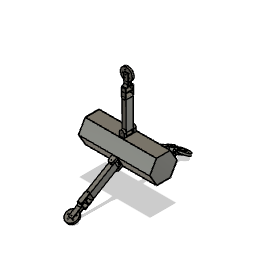
fp1 v5 (Autodesk Fusion 360 design; units mm, degrees)
Autodesk Fusion 360 part; units mm, degrees
sketch "Sketch1" plane through (0, 0, 0) normal (1, 0, 0) x (0, 0, -1)
  line L0 (577.3417, 3.1408) -> (285.9508, 501.563)
  line L1 (285.9508, 501.563) -> (-291.3909, 498.4222)
  line L2 (-291.3909, 498.4222) -> (-577.3417, -3.1408)
  line L3 (-577.3417, -3.1408) -> (-285.9508, -501.563)
  line L4 (-285.9508, -501.563) -> (291.3909, -498.4222)
  line L5 (291.3909, -498.4222) -> (577.3417, 3.1408)
  dimension "d1" = 500
  measures "d1" distance of origin L1
extrude "Extrude1" add sketch "Sketch1" along normal mid plane 3000 makes body 1
copy_body "Body->Comp1" bodies 1 removing the originals makes body 2 in component "old_component"
sketch "Sketch2" plane through (0, 499.9926, 2.72) normal (0, 0.999985, 0.00544) x (1, 0, 0)
  line L0 (-1500, -288.6751) -> (1500, -288.6751)
  line L1 (1500, -288.6751) -> (1500, 288.6751)
  line L2 (1500, 288.6751) -> (-1500, 288.6751)
  line L3 (-1500, 288.6751) -> (-1500, -288.6751)
  line L4 (100, 250) -> (-100, 250)
  line L5 (-100, 250) -> (-100, -250)
  line L6 (-100, -250) -> (100, -250)
  line L7 (100, -250) -> (100, 250)
  line L8 (100, 250) -> (-100, -250) construction
  line L9 (-100, 250) -> (100, -250) construction
  dimension "d4" = 200
  dimension "d5" = 500
  constraint horizontal L4
  constraint perpendicular L4 L5
  constraint parallel L4 L6
  constraint parallel L5 L7
  constraint coincident L8 origin
  constraint coincident L9 origin
  measures "d4" distance of L5.end L6.end
  measures "d5" distance of L4.end L5.end
extrude "Extrude2" add sketch "Sketch2" along normal blind 40 separate body contours L4 L5 L6 L7 makes body 3
sketch "Sketch3" plane through (0, -1.36, 249.9963) normal (0, -0.00544, 0.999985) x (1, 0, 0)
  line L0 (-100, 500) -> (100, 500)
  line L1 (100, 500) -> (100, 540)
  line L2 (100, 540) -> (-100, 540)
  line L3 (-100, 540) -> (-100, 500)
  line L4 (-100, 540) -> (-100, 550)
  line L5 (-100, 550) -> (-100, 650)
  line L6 (100, 540) -> (100, 650)
  circle A0 centre (0, 650) radius 100
  dimension "d8" = 100
  constraint coincident L2.end L3.start
  constraint perpendicular L2 L4
  constraint perpendicular L2 L5
  constraint coincident L1.end L2.start
  constraint perpendicular L2 L6
  constraint coincident L6.end A0
  constraint tangent L6 A0
  measures "d8" distance of L4.end L5.end
extrude "Extrude3" add sketch "Sketch3" against normal blind 500 contours L2 L4 L5 L6 A0 | A0 bodies 3
ref_plane "WorkPlane1" through (0, 624.9908, 3.4) normal (0, 0.00544, -0.999985) x (-1, 0, 0)
sketch "Sketch4" plane through (0, 624.9908, 3.4) normal (0, 0.00544, -0.999985) x (-1, 0, 0)
  arc A0 (100, 25) -> (-100, 25) centre (0, 25) ccw
  line L0 (100, -125) -> (100, 25)
  line L1 (-100, -125) -> (-100, 25)
  line L2 (1500, -125) -> (-1500, -125)
  line L3 (100, -92.0864) -> (-100, -92.0864)
  constraint coincident L0 L3.start
  constraint perpendicular L0 L3
extrude "Extrude4" cut sketch "Sketch4" along normal mid plane 300 contours A0 L0 L1 L3 bodies 3
move_body "Move1" bodies 3 to x (1, 0, 0) y (0, 1, 0) z (0, 0, 1) at (0, 303.2924, 52.7154)
copy_body "Body->Comp2" bodies 3 removing the originals makes body 4 in component "old_component (1)"
sketch "Sketch5" plane through (0, -0.816, 149.9978) normal (0, 0.00544, -0.999985) x (-1, 0, 0)
  arc A0 (100, 650) -> (-100, 650) centre (0, 650) ccw
  line L0 (-100, 650) -> (-100, 532.9136)
  line L1 (-100, 532.9136) -> (100, 532.9136)
  line L2 (100, 532.9136) -> (100, 650)
  line L3 (85, 650) -> (85, 1850)
  arc A1 (85, 1850) -> (-85, 1850) centre (0, 1850) ccw
  line L4 (-85, 1850) -> (-85, 650)
  arc A2 (-85, 650) -> (85, 650) centre (0, 650) ccw
  line L5 (0, 650) -> (0, 1850) construction
  circle A3 centre (0, 650) radius 10
  circle A4 centre (0, 1850) radius 10
  dimension "d18" = 170
  dimension "d19" = 20
  dimension "d20" = 20
  constraint tangent L3 A1
  constraint tangent A1 L4
  constraint parallel L3 L4
  constraint tangent L4 A2
  constraint tangent L3 A2
  constraint vertical L5
  constraint coincident A0.centre A2.centre
  constraint concentric A0 A3
  constraint concentric A1 A4
  measures "d18" diameter of A1
  measures "d19" diameter of A3
  measures "d20" diameter of A4
extrude "Extrude1'" add sketch "Sketch5" along normal blind 300 separate body contours A0 L3 L4 A2 | A0 L3 A1 L4 makes body 5 in component "old_component (2)"
extrude "Extrude1''" cut sketch "Sketch5" along normal blind -120 and the other way blind -550 contours A3 sketch seen with x (1, 0, 0) y (0, 1, 0) z (0, 0, 1) at (0, 303.2924, 52.7154) bodies 4 in component "old_component (1)"
move_body "Move1'" bodies 5 to x (1, 0, 0) y (0, 1, 0) z (0, 0, 1) at (0, 399.9941, 2.176) in component "old_component (2)"
sketch "Sketch6" plane through (-85, 0, 0) normal (-1, 0, 0) x (0, 0, 1)
  line L0 (153.5338, 649.1744) -> (160.0618, 1849.1566)
  line L1 (160.0618, 1849.1566) -> (-139.9337, 1850.7886)
  line L2 (-139.9337, 1850.7886) -> (-146.4618, 650.8064)
  line L3 (-146.4618, 650.8064) -> (153.5338, 649.1744)
  line L4 (-140.075, 1824.8159) -> (-160.0747, 1824.9247)
  line L5 (-160.0747, 1824.9247) -> (-157.7355, 2254.9184)
  line L6 (-137.627, 2274.8093) -> (-127.6271, 2274.7549)
  line L7 (-57.2474, 2344.373) -> (-54.9082, 2774.3667)
  line L8 (-137.7358, 2254.8096) -> (-37.7373, 2254.2655)
  line L9 (-37.7373, 2254.2655) -> (-34.9085, 2774.2579)
  line L10 (-34.9085, 2774.2579) -> (-54.9082, 2774.3667)
  line L11 (159.9206, 1823.1839) -> (179.9203, 1823.0751)
  line L12 (179.9203, 1823.0751) -> (182.2595, 2253.0687)
  line L13 (162.3686, 2273.1772) -> (152.3687, 2273.2316)
  line L14 (82.7506, 2343.6114) -> (85.0898, 2773.6051)
  line L15 (162.2598, 2253.1775) -> (62.2612, 2253.7215)
  line L16 (62.2612, 2253.7215) -> (65.0901, 2773.7139)
  line L17 (65.0901, 2773.7139) -> (85.0898, 2773.6051)
  line L18 (161.4189, 2098.6138) -> (-138.5766, 2100.2458)
  line L19 (-138.6957, 2078.3625) -> (161.2999, 2076.7305)
  line L20 (159.9206, 1823.1839) -> (161.2999, 2076.7305)
  line L21 (161.4189, 2098.6138) -> (162.2598, 2253.1775)
  line L22 (-140.075, 1824.8159) -> (-138.6957, 2078.3625)
  line L23 (-138.5766, 2100.2458) -> (-137.7358, 2254.8096)
  arc A0 (82.7506, 2343.6114) -> (152.3687, 2273.2316) centre (152.7495, 2343.2306) ccw
  arc A1 (-127.6271, 2274.7549) -> (-57.2474, 2344.373) centre (-127.2463, 2344.7538) ccw
  line L24 (182.2595, 2253.0687) -> (162.3686, 2273.1772)
  line L25 (-157.7355, 2254.9184) -> (-137.627, 2274.8093)
  point P0 (-157.6267, 2274.9181)
  point P1 (-57.6282, 2274.3741)
  point P2 (182.3683, 2273.0684)
  point P3 (82.3698, 2273.6124)
  dimension "d47" = 20
  dimension "d48" = 450
  dimension "d49" = 100
  dimension "d50" = 500
  dimension "d52" = 20
  dimension "d53" = 450
  dimension "d54" = 100
  dimension "d55" = 500
  dimension "d57" = 70
  dimension "d58" = 20
  dimension "d59" = 20
  dimension "d60" = 20
  dimension "d61" = 20
  constraint coincident L2 L4.start
  constraint perpendicular L2 L4
  constraint perpendicular L4 L5
  constraint perpendicular L2 L6
  constraint perpendicular L6 L7
  constraint perpendicular L7 L10
  constraint coincident L0 L11.start
  constraint perpendicular L0 L11
  constraint perpendicular L8 L12
  constraint perpendicular L12 L13
  constraint perpendicular L10 L14
  constraint perpendicular L14 L17
  constraint coincident L18.start L20
  constraint coincident L18.end L22
  constraint perpendicular L18 L22
  constraint perpendicular L19 L20
  constraint collinear L20 L21
  constraint collinear L22 L23
  constraint coincident P3 L13
  constraint coincident P3 L14
  constraint tangent L13 A0
  constraint tangent L14 A0
  constraint coincident P1 L6
  constraint coincident P1 L7
  constraint tangent L6 A1
  constraint tangent L7 A1
  constraint equal A0 A1
  constraint coincident P2 L12
  constraint coincident P2 L13
  constraint coincident P0 L5
  constraint coincident P0 L6
  measures "d47" distance of L4.start L4.end
  measures "d48" distance of L4.end P0
  measures "d49" distance of P0 P1
  measures "d50" distance of P1 L7.end
  measures "d52" distance of L11.start L11.end
  measures "d53" distance of L11.end P2
  measures "d54" distance of P2 P3
  measures "d55" distance of P3 L14.end
  measures "d57" radius of A0
  measures "d58" distance of P2 L12.end
  measures "d59" distance of P2 L13.start
  measures "d60" distance of P0 L5.end
  measures "d61" distance of P0 L6.start
ref_plane "WorkPlane2" through (0, 1249.9815, 6.8) normal (0, -0.00544, 0.999985) x (1, 0, 0)
extrude "Extrude1'''" add sketch "Sketch6" against normal blind 170 separate body contours L0 L2 L4 L5 L6 L7 L8 L9 L10 L11 L12 L13 L14 L15 L16 L17 L18 L19 L20 L21 L22 L23 A0 A1 L24 L25 makes body 6 in component "old_component (3)"
sketch "Sketch7" plane through (0, -0.816, 149.9978) normal (0, -0.00544, 0.999985) x (1, 0, 0)
  circle A0 centre (0, 650) radius 10
  circle A1 centre (0, 1850) radius 10
  arc A2 (-85, 650) -> (85, 650) centre (0, 650) ccw
  line L0 (85, 650) -> (85, 1850)
  arc A3 (85, 1850) -> (-85, 1850) centre (0, 1850) ccw
  line L1 (-85, 1850) -> (-85, 650)
  circle A4 centre (0, 1850) radius 10
  constraint concentric A1 A4
extrude "Extrude2'" cut sketch "Sketch7" along normal blind 75 and the other way blind 475 contours A1 A4 bodies 6 in component "old_component (3)"
move_body "Move1''" bodies 6 to x (1, 0, 0) y (0, 1, 0) z (0, 0, 1) at (0, 799.9882, 4.352) in component "old_component (3)"
fillet "Fillet1" radius 65 4 edges at (85, 2624.8585, -145.7228) (-85, 2624.8585, -145.7228) (-85, 2623.1177, 174.2724) (85, 2623.1177, 174.2724) on bodies 6 in component "old_component (3)"
sketch "Sketch8" plane through (0, -0.3808, 69.999) normal (0, -0.00544, 0.999985) x (1, 0, 0)
  line L0 (-85, 2774.0269) -> (-85, 2344.0269)
  line L1 (-85, 2344.0269) -> (85, 2344.0269)
  line L2 (85, 2344.0269) -> (85, 2774.0269)
  line L3 (85, 2774.0269) -> (-85, 2774.0269)
  circle A0 centre (0, 2700) radius 15
  dimension "d74" = 30
  measures "d74" diameter of A0
extrude "Extrude3'" cut sketch "Sketch8" against normal blind 250 contours A0 sketch seen with x (1, 0, 0) y (0, 1, 0) z (0, 0, 1) at (0, 799.9882, 4.352) bodies 6 in component "old_component (3)"
chamfer "Chamfer1" distance 30 angle 45 4 edges at (85, 3573.6476, 79.4419) (-85, 3573.6476, 79.4419) (-85, 3574.3004, -40.5563) (85, 3574.3004, -40.5563) on bodies 6 in component "old_component (3)"
ref_plane "WorkPlane3" through (0, 2558.989, 13.9212) normal (0, 0.00544, -0.999985) x (0, 0.999985, 0.00544)
sketch "Sketch9" plane through (0, 2558.989, 13.9212) normal (0, 0.00544, -0.999985) x (0, 0.999985, 0.00544)
  circle A0 centre (140.9731, 0) radius 15
  circle A1 centre (140.9731, 0) radius 250
  dimension "d78" = 500
  constraint concentric A0 A1
  measures "d78" diameter of A1
extrude "Extrude5" add sketch "Sketch9" along normal mid plane 80 separate body makes body 7
move_body "Move2" bodies 7 to x (1, 0, 0) y (0, 1, 0) z (0, 0, 1) at (20.1861, 274.2541, 1.492)
copy_body "Body->Comp3" bodies 7 removing the originals makes body 8 in component "old_component (4)"
sketch "Sketch10" plane through (0, 0.1632, -29.9996) normal (0, 0.00544, -0.999985) x (-1, 0, 0)
  circle A0 centre (0, 2700) radius 15
  circle A1 centre (0, 2700) radius 250
  circle A2 centre (150, 2700) radius 20
  circle A3 centre (46.3526, 2842.6585) radius 20
  circle A4 centre (-121.3525, 2788.1678) radius 20
  circle A5 centre (-121.3526, 2611.8322) radius 20
  circle A6 centre (46.3525, 2557.3415) radius 20
  dimension "d85" = 40
  dimension "d87" = 360
  measures "d85" diameter of A2
extrude "Extrude1''''" cut sketch "Sketch10" against normal blind 80 contours A2 | A3 | A4 | A5 | A6 sketch seen with x (1, 0, 0) y (0, 1, 0) z (0, 0, 1) at (20.1861, 274.3085, -8.5079) bodies 8 in component "old_component (4)"
shell "Shell1" thickness 20 removed faces 0 bodies 2 in component "old_component"
sketch "Sketch11" plane through (0, 0, 0) normal (1, 0, 0) x (0, 0, -1)
  circle A0 centre (0, 0) radius 2975
  circle A1 centre (0, 0) radius 3225
  dimension "d107" = 250
  dimension "d114" = 5950
  constraint coincident A0.centre A1.centre
  measures "d114" diameter of A0
sketch "Sketch12" plane through (0, 0, 0) normal (0, 1, 0) x (1, 0, 0)
  line L0 (0, 0) -> (-20000, 0)
  line L1 (-20000, 0) -> (-32000, 8000)
  line L2 (-32000, 8000) -> (-44000, 32000)
  line L3 (-44000, 32000) -> (-53796.4742, 69357.7949)
  line L4 (-53796.4742, 69357.7949) -> (-48898.2371, 76705.1506)
  arc A0 (-22003.8966, 81931.1306) -> (-48898.2371, 76705.1506) centre (-32866.5183, 66017.338) ccw
  line L5 (-22003.8966, 81931.1306) -> (27322.2668, 49047.0217)
  line L6 (27322.2668, 49047.0217) -> (88000, 60000)
  line L7 (88000, 60000) -> (146299.1837, 60000)
  constraint coincident L0.start origin
  constraint horizontal L0
  constraint perpendicular L1 L4
  constraint tangent L4 A0
  constraint perpendicular L4 L5
  constraint horizontal L7
copy_body "CopyPasteBodies1" bodies 2 makes body 9 in component "base_link"
copy_body "CopyPasteBodies1'" bodies 4 body 4 seen with x (1, 0, 0) y (0, 1, 0) z (0, 0, 1) at (0, -303.2924, -52.7154) makes body 10 in component "flange_1"
copy_body "CopyPasteBodies1''" bodies 5 body 5 seen with x (1, 0, 0) y (0, 1, 0) z (0, 0, 1) at (0, -399.9941, -2.176) makes body 11 in component "extender_1"
copy_body "CopyPasteBodies1'''" bodies 4 body 4 seen with x (1, 0, 0) y (0, -0.5, 0.866025) z (0, -0.866025, -0.5) at (0, 197.2991, -236.3012) makes body 12 in component "flange_2"
copy_body "CopyPasteBodies1''''" bodies 5 body 5 seen with x (1, 0, 0) y (0, -0.5, 0.866025) z (0, -0.866025, -0.5) at (0, 201.8815, -345.317) makes body 13 in component "extender_2"
copy_body "CopyPasteBodies1'''''" bodies 4 body 4 seen with x (1, 0, 0) y (0, -0.5, -0.866025) z (0, 0.866025, -0.5) at (0, 105.9933, 289.0166) makes body 14 in component "flange_3"
copy_body "CopyPasteBodies1''''''" bodies 5 body 5 seen with x (1, 0, 0) y (0, -0.5, -0.866025) z (0, 0.866025, -0.5) at (0, 198.1126, 347.493) makes body 15 in component "extender_4"
copy_body "CopyPasteBodies1'''''''" bodies 6 body 6 seen with x (1, 0, 0) y (0, 1, 0) z (0, 0, 1) at (0, -799.9882, -4.352) makes body 16 in component "wheel_extender_1"
copy_body "CopyPasteBodies1''''''''" bodies 8 body 8 seen with x (1, 0, 0) y (0, 1, 0) z (0, 0, 1) at (-20.1861, -274.3085, 8.5079) makes body 17 in component "wheel_1"
copy_body "CopyPasteBodies1'''''''''" bodies 6 body 6 seen with x (1, 0, 0) y (0, -0.5, 0.866025) z (0, -0.866025, -0.5) at (0, 403.763, -690.6341) makes body 18 in component "wheel_extender_2"
copy_body "CopyPasteBodies1''''''''''" bodies 6 body 6 seen with x (1, 0, 0) y (0, -0.5, -0.866025) z (0, 0.866025, -0.5) at (0, 396.2251, 694.9861) makes body 19 in component "wheel_extender_4"
copy_body "CopyPasteBodies1'''''''''''" bodies 8 body 8 seen with x (1, 0, 0) y (0, -0.5, 0.866025) z (0, -0.866025, -0.5) at (-20.1861, 147.052, -231.718) makes body 20 in component "wheel_2"
copy_body "CopyPasteBodies1''''''''''''" bodies 8 body 8 seen with x (1, 0, 0) y (0, -0.5, -0.866025) z (0, 0.866025, -0.5) at (-20.1861, 144.5223, 233.3042) makes body 21 in component "wheel_3"
component "old_component" placed x (1, 0, 0) y (0, 1, 0) z (0, 0, 1) at (0, 0, 0)
component "old_component (1)" placed x (1, 0, 0) y (0, 1, 0) z (0, 0, 1) at (0, -303.2924, -52.7154)
component "old_component (2)" placed x (1, 0, 0) y (0, 1, 0) z (0, 0, 1) at (0, -399.9941, -2.176)
component "old_component (1)" placed x (1, 0, 0) y (0, -0.5, 0.866025) z (0, -0.866025, -0.5) at (0, 197.2991, -236.3012)
component "old_component (2)" placed x (1, 0, 0) y (0, -0.5, 0.866025) z (0, -0.866025, -0.5) at (0, 201.8815, -345.317)
component "old_component (1)" placed x (1, 0, 0) y (0, -0.5, -0.866025) z (0, 0.866025, -0.5) at (0, 105.9933, 289.0166)
component "old_component (2)" placed x (1, 0, 0) y (0, -0.5, -0.866025) z (0, 0.866025, -0.5) at (0, 198.1126, 347.493)
component "old_component (3)" placed x (1, 0, 0) y (0, 1, 0) z (0, 0, 1) at (0, -799.9882, -4.352)
component "old_component (4)" placed x (1, 0, 0) y (0, 1, 0) z (0, 0, 1) at (-20.1861, -274.3085, 8.5079)
component "old_component (3)" placed x (1, 0, 0) y (0, -0.5, 0.866025) z (0, -0.866025, -0.5) at (0, 403.763, -690.6341)
component "old_component (3)" placed x (1, 0, 0) y (0, -0.5, -0.866025) z (0, 0.866025, -0.5) at (0, 396.2251, 694.9861)
component "old_component (4)" placed x (1, 0, 0) y (0, -0.5, 0.866025) z (0, -0.866025, -0.5) at (-20.1861, 147.052, -231.718)
component "old_component (4)" placed x (1, 0, 0) y (0, -0.5, -0.866025) z (0, 0.866025, -0.5) at (-20.1861, 144.5223, 233.3042)
component "base_link" placed x (1, 0, 0) y (0, 1, 0) z (0, 0, 1) at (0, 0, 0)
component "flange_1" placed x (1, 0, 0) y (0, 1, 0) z (0, 0, 1) at (0, 0, 0)
component "extender_1" placed x (1, 0, 0) y (0, 1, 0) z (0, 0, 1) at (0, 0, 0)
component "flange_2" placed x (1, 0, 0) y (0, 1, 0) z (0, 0, 1) at (0, 0, 0)
component "extender_2" placed x (1, 0, 0) y (0, 1, 0) z (0, 0, 1) at (0, 0, 0)
component "flange_3" placed x (1, 0, 0) y (0, 1, 0) z (0, 0, 1) at (0, 0, 0)
component "extender_4" placed x (1, 0, 0) y (0, 1, 0) z (0, 0, 1) at (0, 0, 0)
component "wheel_extender_1" placed x (1, 0, 0) y (0, 1, 0) z (0, 0, 1) at (0, 0, 0)
component "wheel_1" placed x (1, 0, 0) y (0, 1, 0) z (0, 0, 1) at (0, 0, 0)
component "wheel_extender_2" placed x (1, 0, 0) y (0, 1, 0) z (0, 0, 1) at (0, 0, 0)
component "wheel_extender_4" placed x (1, 0, 0) y (0, 1, 0) z (0, 0, 1) at (0, 0, 0)
component "wheel_2" placed x (1, 0, 0) y (0, 1, 0) z (0, 0, 1) at (0, 0, 0)
component "wheel_3" placed x (1, 0, 0) y (0, 1, 0) z (0, 0, 1) at (0, 0, 0)
equation "d59 = d58"
equation "d61 = d60"
named bodies: "wheel"
